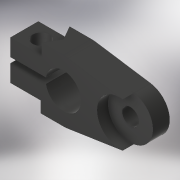
# Autodesk Inventor part: TA08
Saved by Autodesk Inventor 2017 (Build 210142000, 142)
## iProperties
Created: 2019-04-10
Part Number: TA08
Material: ABS Plastic
Document SubType Name: Modeling
Designer: Dell
Density: 1.06 g/cm^3
Appearance: Smooth - Black
Author: Dell
Autodesk Inventor part; units mm, degrees
ref_plane "YZ Plane" through (0, 0, 0) normal (1, 0, 0) x (0, 1, 0)
ref_plane "XZ Plane" through (0, 0, 0) normal (0, 1, 0) x (-1, 0, 0)
ref_plane "XY Plane" through (0, 0, 0) normal (0, 0, 1) x (1, 0, 0)
sketch "Sketch1" plane through (0, 0, 0) normal (0, 0, 1) x (1, 0, 0)
  circle A0 centre (0, 0) radius 3.175
  circle A1 centre (0, 0) radius 5.5
  circle A2 centre (10, 0) radius 4
  line L0 (0.825, 5.4378) -> (10.6, 3.9547)
  line L1 (0.825, -5.4378) -> (10.6, -3.9547)
  circle A3 centre (10, 0) radius 1.5
  dimension "d0" = 6.35
  dimension "d1" = 11
  dimension "d2" = 8
  dimension "d3" = 10
  dimension "d4" = 3
  constraints: 4 centre point, 4 end point, 4 point on circle, 4 tangent, 3 coincident, 1 horizontal alignment
  measures "d0" diameter of A0
  measures "d1" diameter of A1
  measures "d2" diameter of A2
  measures "d3" distance of point (0, 0) A2.centre
  measures "d4" diameter of A3
extrude "Extrusion1" add sketch "Sketch1" along normal blind 5
sketch "Sketch2" plane through (0, 0, 5) normal (0, 0, 1) x (1, 0, 0)
  arc A0 (0.825, 5.4378) -> (0.825, -5.4378) centre (0, 0) ccw projected
  line L0 (0, -5.5) -> (-9.4772, -5.5)
  line L1 (-9.4772, -5.5) -> (-9.4772, -0.5)
  line L2 (-9.4772, -0.5) -> (-5.4772, -0.5)
  line L3 (-5.4772, -0.5) -> (0, -5.5)
  line L4 (0, 5.5) -> (-9.4772, 5.5)
  line L5 (-9.4772, 5.5) -> (-9.4772, 0.5)
  line L6 (-9.4772, 0.5) -> (-5.4772, 0.5)
  line L7 (-5.4772, 0.5) -> (0, 5.5)
  line L8 (-7.4772, -0.5) -> (-7.4772, 0.5) construction
  point P0 (-7.4772, 0)
  dimension "d7" = 1
  dimension "d8" = 4
  constraints: 18 end point, 3 midpoint, 3 perpendicular, 3 point on circle, 2 point on line, 2 tangent, 1 horizontal, 1 horizontal alignment, 1 parallel, 1 vertical alignment
  measures "d7" distance between parallel lines of L2 L6
  measures "d8" distance of L1.end L2.end
extrude "Extrusion2" add sketch "Sketch2" against normal blind 5 contours L7 A0 | A0 L6 L5 L4 | A0 L0 L1 L2
sketch "Sketch3" plane through (-9.4772, -5.5, 5) normal (0, -1, 0) x (1, 0, 0)
  line L0 (0, 0) -> (4, 0) construction
  line L1 (0, 0) -> (0, -5) construction
  line L2 (4, -5) -> (0, -5) construction
  line L3 (4, 0) -> (4, -5) construction
  line L4 (0, 0) -> (4, 0) construction
  line L5 (2, 0) -> (2, -5) construction
  circle A0 centre (3, -2.5) radius 1.5
  point P0 (9.4772, -5)
  point P1 (2, -2.5)
  dimension "d11" = 3
  dimension "d12" = 1
  constraints: 3 midpoint, 2 end point, 1 centre point, 1 horizontal alignment
  measures "d11" diameter of A0
  measures "d12" distance from line of L5 A0.centre
extrude "Extrusion3" cut sketch "Sketch3" against normal through all
sketch "Sketch4" plane through (0, 0, 5) normal (0, 0, 1) x (1, 0, 0)
  line L0 (-9.4772, 0.5) -> (0, 0.5)
  line L1 (0, 0.5) -> (0, -0.5)
  line L2 (0, -0.5) -> (-9.4772, -0.5)
  line L3 (-9.4772, -0.5) -> (-9.4772, 0.5)
  point P0 (0, 0)
  point P1 (0, 0)
  constraints: 8 end point, 2 coincident, 2 parallel, 1 horizontal, 1 midpoint, 1 perpendicular
extrude "Extrusion4" cut sketch "Sketch4" against normal through all
sketch "Sketch5" plane through (-9.4772, 5.5, 5) normal (0, 1, 0) x (1, 0, 0)
  circle A0 centre (3, 2.5) radius 1.5 projected
  line L0 (7.0415, 2.5) -> (5.0207, -1)
  line L1 (5.0207, -1) -> (0.9793, -1)
  line L2 (0.9793, -1) -> (-1.0415, 2.5)
  line L3 (-1.0415, 2.5) -> (0.9793, 6)
  line L4 (0.9793, 6) -> (5.0207, 6)
  line L5 (5.0207, 6) -> (7.0415, 2.5)
  point P0 (9.4772, 5)
  dimension "d17" = 7
  constraints: 12 end point, 1 coincident, 1 horizontal alignment, 13 other
  measures "d17" distance between parallel lines of L1 L4
extrude "Extrusion5" cut sketch "Sketch5" against normal blind 2 contours A0 | L0 L1 L2 L3 L4 L5
sketch "Sketch6" plane through (-9.4772, -5.5, 5) normal (0, -1, 0) x (1, 0, 0)
  circle A0 centre (3, -2.5) radius 1.5 projected
  circle A1 centre (3, -2.5) radius 3.5
  point P0 (9.4772, -5)
  dimension "d20" = 7
  constraints: 1 centre point, 1 coincident
  measures "d20" diameter of A1
extrude "Extrusion6" cut sketch "Sketch6" against normal blind 2 contours A0 | A1
sketch "Sketch7" plane through (0, 0, 5) normal (0, 0, 1) x (1, 0, 0)
  circle A0 centre (10, 0) radius 1.5 projected
  arc A1 (10.6, -3.9547) -> (10.6, 3.9547) centre (10, 0) ccw projected
  circle A2 centre (10, 0) radius 4
  point P0 (0, 0)
  constraints: 1 coincident, 3 other
extrude "Extrusion7" cut sketch "Sketch7" against normal blind 2
sketch "Sketch8" plane through (-9.4772, -3.5, 5) normal (0, -1, 0) x (1, 0, 0)
  line L0 (5.4495, -5) -> (0.5505, -5) projected
  line L1 (0, 0) -> (0, -5) projected
  line L2 (3, -5) -> (0, -5)
  line L3 (0, -5) -> (0, 0)
  line L4 (0, 0) -> (3, 0)
  line L5 (3, 0) -> (3, -5)
  point P0 (9.4772, -5)
  constraints: 8 end point, 2 parallel, 1 horizontal, 1 midpoint, 1 perpendicular
extrude "Extrusion8" cut sketch "Sketch8" along normal through all
sketch "Sketch9" plane through (-9.4772, 3.5, 5) normal (0, 1, 0) x (1, 0, 0)
  circle A0 centre (3, 2.5) radius 1.5 projected
  line L0 (5.5981, 0) -> (0.4019, 0) projected
  line L1 (0, 0) -> (0, 5) projected
  line L2 (3, 0) -> (0, 0)
  line L3 (0, 0) -> (0, 5)
  line L4 (0, 5) -> (3, 5)
  line L5 (3, 5) -> (3, 0)
  point P0 (9.4772, 5)
  constraints: 8 end point, 2 parallel, 1 horizontal, 1 midpoint, 1 perpendicular
extrude "Extrusion9" cut sketch "Sketch9" along normal through all contours L5 A0 | A0 L5 L0 L2 L1 L4 picked at (2.8803, 2.0145)
body "Solid1"
